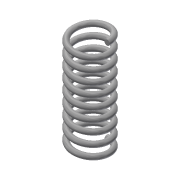
# Autodesk Inventor part: PP-07
Saved by Autodesk Inventor 2022 (Build 260148000, 148)
## iProperties
Created: 2008-09-23
Part Number: PP-07
Document SubType Name: Modeling
Designer: Mark Flayler
Mass: 0.143514 g
Surface Area: 1.4683 cm^2
Volume: 0.0182588 cm^3
Density: 7.86 g/cm^3
Material: Steel, Mild
Description: SPRING
Appearance: Steel
Author: Mark Flayler
Autodesk Inventor part; units mm, degrees
ref_plane "YZ Plane" through (0, 0, 0) normal (1, 0, 0) x (0, 1, 0)
ref_plane "XZ Plane" through (0, 0, 0) normal (0, 1, 0) x (-1, 0, 0)
ref_plane "XY Plane" through (0, 0, 0) normal (0, 0, 1) x (1, 0, 0)
sketch "Sketch1" plane through (0, 0, 0) normal (0, 0, 1) x (1, 0, 0)
  circle A0 centre (0, 0) radius 1.85 construction
  dimension "d0" = 3.7
  constraints: 1 centre point, 1 coincident
  measures "d0" diameter of A0
sketch "Sketch2" plane through (0, 0, 0) normal (0, 1, 0) x (-1, 0, 0)
  line L0 (1.85, 0) -> (-1.85, 0) construction
  circle A0 centre (-1.6, 0) radius 0.25
  point P0 (0, 0)
  dimension "d1" = 0.5
  constraints: 2 horizontal alignment, 2 other
coil "Coil1" sketch "Sketch2" operation add axis through (0, 0, -10) along (0, 0, -1) pitch 1.0054 turns 9.25 hand left
body "Solid1"
